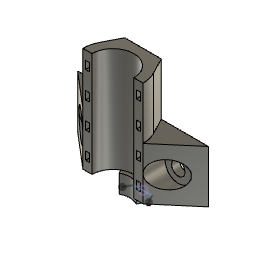
Frame-cable-locker v5 (Autodesk Fusion 360 design; units mm, degrees)
Autodesk Fusion 360 part; units mm, degrees
sketch "Sketch10" plane through (0, 0, 0) normal (0, 1, 0) x (1, 0, 0)
  line L0 (0, 0) -> (8, 0)
  line L1 (8, 0) -> (11.5, 0)
  line L2 (11.5, 0) -> (11.5, -40)
  line L3 (11.5, -40) -> (8, -40)
  line L4 (8, -40) -> (8, 0)
  line L5 (8, 0) -> (9, 0)
  line L6 (9, 0) -> (9, -3.5) construction
  line L7 (9, -3.5) -> (10.5, -3.5)
  line L8 (10.5, -3.5) -> (10.5, -6.5)
  line L9 (10.5, -6.5) -> (9, -6.5)
  line L10 (9, -6.5) -> (9, -3.5)
  line L11 (9, -6.5) -> (9, -13.5) construction
  line L12 (9, -13.5) -> (10.5, -13.5)
  line L13 (10.5, -13.5) -> (10.5, -16.5)
  line L14 (10.5, -16.5) -> (9, -16.5)
  line L15 (9, -16.5) -> (9, -13.5)
  line L16 (9, -16.5) -> (9, -23.5) construction
  line L17 (9, -23.5) -> (10.5, -23.5)
  line L18 (10.5, -23.5) -> (10.5, -26.5)
  line L19 (10.5, -26.5) -> (9, -26.5)
  line L20 (9, -26.5) -> (9, -23.5)
  line L21 (9, -26.5) -> (9, -33.5) construction
  line L22 (9, -33.5) -> (10.5, -33.5)
  line L23 (10.5, -33.5) -> (10.5, -36.5)
  line L24 (10.5, -36.5) -> (9, -36.5)
  line L25 (9, -36.5) -> (9, -33.5)
  dimension "d105" = 8
  dimension "d106" = 3.5
  dimension "d107" = 40
  dimension "d108" = 3.5
  dimension "d109" = 1
  dimension "d110" = 3.5
  dimension "d111" = 1.5
  dimension "d112" = 3
  dimension "d113" = 1.5
  dimension "d114" = 7
  dimension "d115" = 1.5
  dimension "d116" = 3
  dimension "d117" = 1.5
  dimension "d118" = 7
  dimension "d119" = 1.5
  dimension "d120" = 3
  dimension "d161" = 7
  dimension "d162" = 1.5
  dimension "d163" = 3
  constraint coincident L0.start origin
  constraint horizontal L0
  constraint parallel L0 L1
  constraint vertical L2
  constraint perpendicular L2 L3
  constraint perpendicular L4 L5
  constraint perpendicular L5 L6
  constraint perpendicular L6 L7
  constraint perpendicular L7 L8
  constraint perpendicular L8 L9
  constraint perpendicular L9 L11
  constraint perpendicular L11 L12
  constraint perpendicular L12 L13
  constraint perpendicular L13 L14
  constraint perpendicular L14 L16
  constraint horizontal L17
  constraint vertical L18
  constraint horizontal L19
  constraint vertical L20
  constraint perpendicular L19 L21
  constraint horizontal L22
  constraint vertical L23
  constraint horizontal L24
  constraint vertical L25
  measures "d105" distance of L0.start L0.end
  measures "d106" distance of L0.end L1.end
  measures "d107" distance of L1.end L2.end
  measures "d108" distance of L2.end L3.end
  measures "d109" distance of L0.end L5.end
  measures "d110" distance of L5.end L6.end
  measures "d111" distance of L6.end L7.end
  measures "d112" distance of L7.end L8.end
  measures "d113" distance of L8.end L9.end
  measures "d114" distance of L9.end L11.end
  measures "d115" distance of L11.end L12.end
  measures "d116" distance of L12.end L13.end
  measures "d117" distance of L13.end L14.end
  measures "d118" distance of L14.end L16.end
  measures "d119" distance of L16.end L17.end
  measures "d120" distance of L16.end L19.end
  measures "d161" distance of L19.end L21.end
  measures "d162" distance of L21.end L22.end
  measures "d163" distance of L21.end L24.end
revolve "Revolve3" add sketch "Sketch10" angle 180 about axis through (0, 0, 1.75) along (0, 0, 1) contours L1 L2 L3 L4 L5 | L22 L23 L24 L25
sketch "Sketch12" plane through (0, 0, 0) normal (0, 0, -1) x (1, 0, 0)
  line L0 (11.5, 0) -> (8, 0)
  arc A0 (-8, 0) -> (8, 0) centre (0, 0) ccw
  line L1 (-8, 0) -> (-11.5, 0)
  arc A1 (-11.5, 0) -> (11.5, 0) centre (0, 0) ccw
  line L2 (0, 0) -> (0, -11.5)
  line L3 (0, -11.5) -> (-25, -11.5)
  line L4 (-25, -11.5) -> (-11.5, 0)
  line L5 (0, -11.5) -> (25, -11.5)
  line L6 (11.5, 0) -> (25, -11.5)
  dimension "d125" = 25
  dimension "d126" = 25
  constraint coincident A0.centre A1.centre
  constraint midpoint A1 L2.end
  constraint perpendicular L2 L3
  constraint coincident L1.end A1.start
  constraint tangent A1 L5
  constraint perpendicular L2 L5
  constraint coincident L0.start A1.end
  measures "d125" distance of L2.end L3.end
  measures "d126" distance of L2.end L5.end
extrude "Extrude6" add sketch "Sketch12" against normal blind 20 contours A1 L5 L6 | A1 L3 L4
sketch "Sketch13" plane through (0, 0, 40) normal (0, 0, 1) x (-1, 0, 0)
  line L0 (-8, 0) -> (-11.5, 0)
  arc A0 (-11.5, 0) -> (11.5, 0) centre (0, 0) ccw
  line L1 (11.5, 0) -> (8, 0)
  arc A1 (-8, 0) -> (8, 0) centre (0, 0) ccw
  line L2 (0, 0) -> (0, -11.5) construction
  line L3 (0, -11.5) -> (7, -11.5)
  line L4 (7, -11.5) -> (10.2152, -5.2821)
  line L5 (0, -11.5) -> (-7, -11.5)
  line L6 (-7, -11.5) -> (-10.2152, -5.2821)
  dimension "d129" = 7
  dimension "d130" = 7
  constraint coincident A0.centre A1.centre
  constraint midpoint A0 L2.end
  constraint perpendicular L2 L3
  constraint coincident A0 L4.end
  constraint tangent A0 L4
  constraint perpendicular L2 L5
  constraint coincident A0 L6.end
  constraint tangent A0 L6
  measures "d129" distance of L2.end L3.end
  measures "d130" distance of L2.end L5.end
extrude "Extrude7" add sketch "Sketch13" against normal blind 20 contours A0 L5 L6 | A0 L3 L4
sketch "Sketch18" plane through (0, 11.5, 0) normal (0, 1, 0) x (-1, 0, 0)
  line L0 (-25, 0) -> (25, 0)
  line L1 (25, 0) -> (25, 20)
  line L2 (25, 20) -> (7, 20)
  line L3 (-7, 20) -> (-25, 20)
  line L4 (-25, 20) -> (-25, 0)
  line L5 (0, 0) -> (-16.5, 0) construction
  line L6 (-16.5, 0) -> (-16.5, 10) construction
  circle A0 centre (-16.5, 10) radius 2.6
  circle A1 centre (-16.5, 10) radius 5
  line L7 (0, 0) -> (16.5, 0) construction
  line L8 (16.5, 0) -> (16.5, 10) construction
  circle A2 centre (16.5, 10) radius 2.6
  circle A3 centre (16.5, 10) radius 5
  line L9 (7, 20) -> (7, 40)
  line L10 (7, 40) -> (-7, 40)
  line L11 (-7, 40) -> (-7, 20)
  dimension "d143" = 16.5
  dimension "d144" = 10
  dimension "d145" = 5.2
  dimension "d146" = 10
  dimension "d152" = 16.5
  dimension "d153" = 10
  dimension "d154" = 5.2
  dimension "d155" = 10
  constraint coincident L5.start L7.start
  constraint parallel L0 L5
  constraint vertical L6
  constraint coincident L6.end A0.centre
  constraint concentric A0 A1
  constraint parallel L0 L7
  constraint perpendicular L7 L8
  constraint coincident L8.end A2.centre
  constraint concentric A2 A3
  measures "d143" distance of L5.start L5.end
  measures "d144" distance of L5.end L6.end
  measures "d145" diameter of A0
  measures "d146" diameter of A1
  measures "d152" distance of L5.start L7.end
  measures "d153" distance of L7.end L8.end
  measures "d154" diameter of A2
  measures "d155" diameter of A3
extrude "Extrude9" cut sketch "Sketch18" against normal blind 3 contours A0
extrude "Extrude10" cut sketch "Sketch18" against normal blind 10 from surface at -3 contours A0 | A1
extrude "Extrude11" cut sketch "Sketch18" against normal blind 3 contours A2
extrude "Extrude12" cut sketch "Sketch18" against normal blind 10 from surface at -3 contours A2 | A3
revolve "Revolve4" cut sketch "Sketch10" angle 360 about axis through (0, 0, 1.75) along (0, 0, 1) contours L22 L23 L24 L25
sketch "Sketch19" plane through (0, 0, 0) normal (0, 1, 0) x (1, 0, 0)
  line L0 (7.5, 2) -> (9, 2)
  line L1 (9, 2) -> (9, 5)
  line L2 (9, 5) -> (7.5, 5)
  line L3 (7.5, 5) -> (7.5, 2)
  line L4 (6.5, 0) -> (10, 0)
  line L5 (10, 0) -> (10, 7)
  line L6 (10, 7) -> (6.5, 7)
  line L7 (6.5, 7) -> (6.5, 0)
  dimension "d165" = 3
  dimension "d166" = 1.5
  dimension "d167" = 1
  dimension "d168" = 1
  dimension "d169" = 2
  dimension "d170" = 2
  dimension "d171" = 6.5
  constraint horizontal L0
  constraint vertical L1
  constraint horizontal L2
  constraint vertical L3
  constraint horizontal L4
  constraint vertical L5
  constraint horizontal L6
  constraint vertical L7
  constraint coincident L4 origin
  measures "d165" distance of L0.end L1.end
  measures "d166" distance of L1.end L2.end
  measures "d167" distance of L3 L7
  measures "d168" distance of L1 L5
  measures "d169" distance of L0 L4
  measures "d170" distance of L2 L6
  measures "d171" distance of origin L7
revolve "Revolve5" add sketch "Sketch19" angle 120 about axis through (0, 0, 1.75) along (0, 0, 1) second angle -60
sketch "Sketch20" plane through (0, 0, -7) normal (0, 0, -1) x (1, 0, 0)
  line L0 (5, -8.6603) -> (3.25, -5.6292)
  arc A0 (-3.25, -5.6292) -> (3.25, -5.6292) centre (0, 0) ccw
  line L1 (-3.25, -5.6292) -> (-5, -8.6603)
  arc A1 (-5, -8.6603) -> (5, -8.6603) centre (0, 0) ccw
  line L2 (-5, -8.6603) -> (-3.5, -11.5)
  line L3 (5, -8.6603) -> (3.5, -11.5)
  line L4 (-3.5, -11.5) -> (3.5, -11.5)
  point P0 (0, -11.5)
  dimension "d179" = 122.156
  dimension "d182" = 11.5
  dimension "d183" = 117.844
  dimension "d186" = 117.844
  constraint coincident L1.end A1.start
  constraint coincident L0.start A1.end
  measures "d179" angle of L1 L2
  measures "d182" distance of A0.centre L4
  measures "d183" angle of L2 L4
  measures "d186" angle of L3 L4
extrude "Extrude14" add sketch "Sketch20" against normal blind 7 contours A1 L2 L3 L4
extrude "Extrude13" [suppressed]
